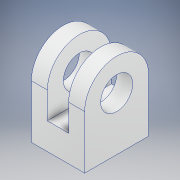
# Autodesk Inventor part: Gripper_Link_Holder
Saved by Autodesk Inventor 2021.3 (Build 253353000, 353)
## iProperties
Created: 2021-04-16
Part Number: Gripper_Link_Holder
Material: Aluminum 6061
Document SubType Name: Modeling
Designer: domin
Density: 2.7 g/cm^3
Appearance: Aluminum - Flat
Mass: 2.98593 g
Surface Area: 10.5642 cm^2
Volume: 1.1059 cm^3
Author: domin
Autodesk Inventor part; units mm, degrees
ref_plane "YZ Plane" through (0, 0, 0) normal (1, 0, 0) x (0, 1, 0)
ref_plane "XZ Plane" through (0, 0, 0) normal (0, 1, 0) x (-1, 0, 0)
ref_plane "XY Plane" through (0, 0, 0) normal (0, 0, 1) x (1, 0, 0)
sketch "Sketch1" plane through (0, 0, 0) normal (0, 0, 1) x (1, 0, 0)
  line L0 (-5, 0) -> (5, 0)
  line L1 (5, 0) -> (5, 16)
  line L2 (5, 16) -> (-5, 16)
  line L3 (-5, 16) -> (-5, 0)
  point P0 (0, 0)
  dimension "d0" = 0
  dimension "d1" = 10
  dimension "d2" = 16
  dimension "d3" = 5
  constraints: 8 end point, 2 parallel, 1 horizontal, 1 perpendicular
  measures "d0" distance from line of point (0, 0) L0
  measures "d1" distance between parallel lines of L1 L3
  measures "d2" distance between parallel lines of L0 L2
  measures "d3" distance from line of point (0, 0) L3
extrude "Extrusion1" add sketch "Sketch1" along normal mid plane 12
sketch "Sketch2" plane through (0, 0, 6) normal (0, 0, 1) x (1, 0, 0)
  line L0 (5, 16) -> (-5, 16) projected
  line L1 (-2, 16) -> (2, 16)
  line L2 (2, 16) -> (2, 5)
  line L3 (2, 5) -> (-2, 5)
  line L4 (-2, 5) -> (-2, 16)
  point P0 (0, 0)
  dimension "d6" = 11
  dimension "d7" = 4
  dimension "d8" = 2
  constraints: 8 end point, 2 parallel, 1 horizontal, 1 perpendicular, 1 point on line
  measures "d6" distance of L3.end L1.start
  measures "d7" distance between parallel lines of L2 L4
  measures "d8" distance from line of point (0, 0) L4
extrude "Extrusion2" cut sketch "Sketch2" against normal through all
sketch "Sketch3" plane through (5, 0, 6) normal (1, 0, 0) x (0, 0, -1)
  circle A0 centre (6, 10) radius 3
  line L0 (0, 0) -> (12, 0) projected
  line L1 (12, 16) -> (0, 16) projected
  point P0 (6, 0)
  point P1 (6, 0)
  dimension "d11" = 6
  dimension "d12" = 6
  constraints: 1 centre point, 1 midpoint, 1 vertical alignment
  measures "d11" distance from line of A0.centre L1
  measures "d12" diameter of A0
hole "Hole1" at (5, 10, 0) direction (-1, 0, 0) diameter 6 end through all
fillet "Fillet1" radius 6 4 edges at (3.5, 16, 6) (3.5, 16, -6) (-3.5, 16, -6) (-3.5, 16, 6)
sketch "Sketch4" plane through (-5, 0, 6) normal (0, -1, 0) x (1, 0, 0)
  circle A0 centre (5, -6) radius 1.5
  dimension "d21" = 3
  constraints: 1 centre point, 1 coincident
  measures "d21" diameter of A0
hole "Hole2" at (0, 0, 0) direction (0, 1, 0) diameter 2.459 depth 5 thread size "M3x0.5" class "6H" standard "ISO Metric profile"
equation "\"d3\" = 0.5 * d1"
equation "\"d8\" = 0.5 * d7"
equation "\"d13\" = d12"
body "Solid1"
